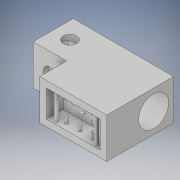
# Autodesk Inventor part: 20190425_NewHolde3
Saved by Autodesk Inventor 2018 (Build 220112000, 112)
## iProperties
Created: 2019-04-24
Part Number: 20190425_NewHolde3
Material: Generic
Document SubType Name: Modeling
Designer: 120pa
Density: 1 g/cm^3
Appearance: Default
Author: 120pa
Autodesk Inventor part; units mm, degrees
ref_plane "YZ Plane" through (0, 0, 0) normal (1, 0, 0) x (0, 1, 0)
ref_plane "XZ Plane" through (0, 0, 0) normal (0, 1, 0) x (-1, 0, 0)
ref_plane "XY Plane" through (0, 0, 0) normal (0, 0, 1) x (1, 0, 0)
sketch "Sketch1" plane through (0, 0, 0) normal (0, 0, 1) x (1, 0, 0)
  line L0 (0, 0) -> (10, 0)
  line L1 (10, 0) -> (10, 6)
  line L2 (10, 6) -> (0, 6)
  line L3 (0, 6) -> (0, 0)
  dimension "d0" = 10
  dimension "d1" = 6
  constraints: 8 end point, 2 parallel, 1 horizontal, 1 perpendicular
  measures "d0" distance of L2.end L1.end
  measures "d1" distance of L1.end L0.end
extrude "Extrusion1" add sketch "Sketch1" along normal blind 4
sketch "Sketch2" plane through (0, 0, 4) normal (0, 0, 1) x (1, 0, 0)
  line L0 (1, 1) -> (9, 1)
  line L1 (9, 1) -> (9, 5)
  line L2 (9, 5) -> (1, 5)
  line L3 (1, 5) -> (1, 1)
  point P0 (0, 0)
  dimension "d4" = 8
  dimension "d5" = 4
  constraints: 8 end point, 2 parallel, 1 horizontal, 1 perpendicular
  measures "d4" distance of L2.end L1.end
  measures "d5" distance of L1.end L0.end
extrude "Extrusion2" cut sketch "Sketch2" against normal blind 2.5
sketch "Sketch5" plane through (1, 1, 4) normal (0, 1, 0) x (1, 0, 0)
  circle A0 centre (1, 0.5) radius 0.25
  point P0 (-1, 4)
  dimension "d14" = 0.5
  constraints: 1 centre point
  measures "d14" diameter of A0
sketch "Sketch6" plane through (1, 1, 4) normal (0, 1, 0) x (1, 0, 0)
  circle A0 centre (7, 0.5) radius 0.25
  point P0 (-1, 4)
  dimension "d15" = 0.5
  constraints: 1 centre point
  measures "d15" diameter of A0
extrude "Extrusion4" add sketch "Sketch5" along normal blind 4
extrude "Extrusion5" add sketch "Sketch6" along normal blind 4
sketch "Sketch14" plane through (0, 0, 0) normal (0, 0, -1) x (-1, 0, 0)
  line L0 (0, 6) -> (0, 0) projected
  line L1 (0, 0) -> (-10, 0) projected
  line L2 (0, 6) -> (-10, 6)
  line L3 (-10, 6) -> (-10, 0)
  line L4 (-10, 0) -> (0, 0)
  line L5 (0, 0) -> (0, 6)
  constraints: 8 end point, 2 parallel, 1 horizontal, 1 perpendicular
extrude "Extrusion12" add sketch "Sketch14" along normal blind 6
sketch "Sketch15" plane through (0, 0, 4) normal (-1, 0, 0) x (0, 0, 1)
  line L0 (-10, 0) -> (0, 0) projected
  line L1 (-10, 0) -> (-4, 0)
  line L2 (-4, 0) -> (-4, 6)
  line L3 (-4, 6) -> (-10, 6)
  line L4 (-10, 6) -> (-10, 0)
  point P0 (-4, 0)
  dimension "d42" = 6
  dimension "d43" = 6
  constraints: 8 end point, 2 parallel, 1 horizontal, 1 perpendicular
  measures "d42" distance of L3.end L2.end
  measures "d43" distance of L2.end L1.end
extrude "Extrusion13" add sketch "Sketch15" along normal blind 5
sketch "Sketch16" plane through (-5, 0, 4) normal (-1, 0, 0) x (0, 0, 1)
  circle A0 centre (-7, 3) radius 2.25
  point P0 (-4, 0)
  dimension "d46" = 4.5
  constraints: 1 centre point
  measures "d46" diameter of A0
extrude "Extrusion14" cut sketch "Sketch16" against normal blind 15
sketch "Sketch17" plane through (0, 0, 1.5) normal (0, 0, 1) x (1, 0, 0)
  circle A0 centre (3, 3) radius 0.25
  point P0 (0, 0)
  dimension "d49" = 0.5
  constraints: 1 centre point
  measures "d49" diameter of A0
extrude "Extrusion15" add sketch "Sketch17" along normal blind 0.5
sketch "Sketch18" plane through (0, 0, 1.5) normal (0, 0, 1) x (1, 0, 0)
  circle A0 centre (5, 3) radius 0.25
  circle A1 centre (7, 3) radius 0.25
  circle A2 centre (4, 4) radius 0.25
  circle A3 centre (6, 4) radius 0.25
  circle A4 centre (4, 2) radius 0.25
  circle A5 centre (6, 2) radius 0.25
  point P0 (0, 0)
  dimension "d52" = 0.5
  dimension "d53" = 0.5
  dimension "d54" = 0.5
  dimension "d55" = 0.5
  dimension "d56" = 0.5
  dimension "d57" = 0.5
  constraints: 6 centre point
  measures "d52" diameter of A0
  measures "d53" diameter of A1
  measures "d54" diameter of A2
  measures "d55" diameter of A3
  measures "d56" diameter of A4
  measures "d57" diameter of A5
extrude "Extrusion16" add sketch "Sketch18" along normal blind 0.5
sketch "Sketch19" plane through (1, 1, 4) normal (0, 1, 0) x (1, 0, 0)
  point P0 (-1, 4)
sketch "Sketch20" plane through (1, 1, 4) normal (0, 1, 0) x (1, 0, 0)
  circle A0 centre (2, 1) radius 0.25
  circle A1 centre (4, 1) radius 0.25
  circle A2 centre (6, 1) radius 0.25
  point P0 (-1, 4)
  dimension "d60" = 0.5
  dimension "d61" = 0.5
  dimension "d62" = 0.5
  constraints: 3 centre point
  measures "d60" diameter of A0
  measures "d61" diameter of A1
  measures "d62" diameter of A2
extrude "Extrusion17" add sketch "Sketch20" along normal blind 0.8
sketch "Sketch21" plane through (1, 5, 4) normal (0, -1, 0) x (1, 0, 0)
  circle A0 centre (2, -1) radius 0.25
  circle A1 centre (4, -1) radius 0.25
  circle A2 centre (6, -1) radius 0.25
  point P0 (-1, -4)
  dimension "d65" = 0.5
  dimension "d66" = 0.5
  dimension "d67" = 0.5
  constraints: 3 centre point
  measures "d65" diameter of A0
  measures "d66" diameter of A1
  measures "d67" diameter of A2
extrude "Extrusion18" add sketch "Sketch21" along normal blind 0.8
sketch "Sketch22" plane through (0, 0, 0) normal (0, 0, 1) x (1, 0, 0)
  circle A0 centre (-2.5, 3) radius 1
  point P0 (0, 0)
  dimension "d70" = 2
  constraints: 1 centre point
  measures "d70" diameter of A0
extrude "Extrusion19" cut sketch "Sketch22" against normal blind 6
sketch "Sketch23" plane through (0, 0, 4) normal (0, -1, 0) x (1, 0, 0)
  point P0 (0, -4)
sketch "Sketch24" plane through (0, 0, 4) normal (0, -1, 0) x (1, 0, 0)
  circle A0 centre (-2.5, -7) radius 1
  point P0 (0, -4)
  dimension "d73" = 2
  constraints: 1 centre point
  measures "d73" diameter of A0
extrude "Extrusion20" cut sketch "Sketch24" against normal blind 6
body "Solid1"
